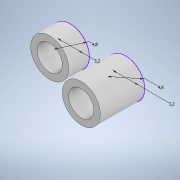
# Autodesk Inventor part: spacer_v1
Saved by Autodesk Inventor 2022 (Build 260153000, 153)
## iProperties
Created: 2021-08-30
Part Number: spacer_v1
Material: Generic
Document SubType Name: Modeling
Designer: jonar
Density: 1 g/cm^3
Appearance: Default
Author: jonar
Autodesk Inventor part; units mm, degrees
ref_plane "YZ Plane" through (0, 0, 0) normal (1, 0, 0) x (0, 1, 0)
ref_plane "XZ Plane" through (0, 0, 0) normal (0, 1, 0) x (-1, 0, 0)
ref_plane "XY Plane" through (0, 0, 0) normal (0, 0, 1) x (1, 0, 0)
sketch "Sketch1" plane through (0, 0, 0) normal (0, 0, 1) x (1, 0, 0)
  circle A0 centre (-6, 4) radius 1.6
  circle A1 centre (-6, 4) radius 2.4
  circle A2 centre (-13, 4) radius 1.6
  circle A3 centre (-13, 4) radius 2.4
  point P0 (0, 0)
  dimension "d0" = 3.2
  dimension "d1" = 4.8
  dimension "d2" = 3.2
  dimension "d3" = 4.8
  constraints: 4 centre point, 2 coincident
  measures "d0" diameter of A0
  measures "d1" diameter of A1
  measures "d2" diameter of A2
  measures "d3" diameter of A3
extrude "Extrusion1" add sketch "Sketch1" along normal blind 2.6 contours A3
extrude "Extrusion2" add sketch "Sketch1" along normal blind 5.6 contours A1
body "Solid1"
